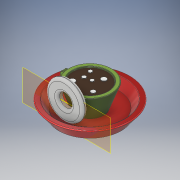
# Autodesk Inventor part: cup
Saved by Autodesk Inventor 2017 (Build 210142000, 142)
## iProperties
Created: 2018-09-11
Part Number: cup
Material: Generic
Document SubType Name: Modeling
Designer: qthuynh
Density: 1 g/cm^3
Appearance: Default
Author: qthuynh
Autodesk Inventor part; units mm, degrees
ref_plane "YZ Plane" through (0, 0, 0) normal (1, 0, 0) x (0, 1, 0)
sketch "Sketch1" plane through (0, 0, 0) normal (0, 0, 1) x (1, 0, 0)
  line L0 (0, 0) -> (0, 101.6)
  line L1 (0, 101.6) -> (61.7893, 101.6)
  line L2 (61.7893, 101.6) -> (88.5597, 137.6833)
  line L3 (88.5597, 137.6833) -> (109.1155, 137.6833)
  line L4 (109.1155, 137.6833) -> (67.5258, 23.4311)
  line L5 (67.5258, 23.4311) -> (143.0565, 23.4311)
  line L6 (143.0565, 23.4311) -> (172.2256, 62.7476)
  line L7 (172.2256, 62.7476) -> (199.4655, 62.7476)
  line L8 (199.4655, 62.7476) -> (152.9127, 0)
  line L9 (152.9127, 0) -> (0, 0)
  dimension "d0" = 101.6
  constraints: 20 end point, 6 parallel, 1 perpendicular, 1 vertical
  measures "d0" distance of L0.start L0.end
revolve "Revolution1" add sketch "Sketch1" angle 360 about axis through (0, 0, 0) along (0, 1, 0)
fillet "Fillet1" radius 3.175 5 edges at (-172.2256, 62.7476, 0) (-152.9127, 0, 0) (-199.4655, 62.7476, 0) (-109.1155, 137.6833, 0) (-88.5597, 137.6833, 0)
ref_plane "Work Plane2" through (0, 0, 0) normal (0, 0, 1) x (1, 0, 0)
sketch "Sketch5" plane through (0, 0, 0) normal (0, 0, 1) x (1, 0, 0)
  ellipse E0 centre (-83.3046, 79.9703) end of major axis (-133.0665, 118.4759) minor radius 30.4237
  ellipse E1 centre (-83.3046, 79.9703) end of major axis (-114.3425, 103.9873) minor radius 19.8321
  point P0 (0, 0)
  constraints: 1 coincident, 4 other
extrude "Extrusion2" add sketch "Sketch5" along normal mid plane 25.4
fillet "Fillet2" radius 3.175 8 edges at (-121.3784, 124.9012, 12.7) (-123.4885, 77.2986, 12.7) (-121.3784, 124.9012, -12.7) (-123.4885, 77.2986, -12.7) (-107.6722, 108.0804, 12.7) (-109.1356, 78.1235, 12.7) (-107.6722, 108.0804, -12.7) (-109.1356, 78.1235, -12.7)
ref_plane "Work Plane3" through (0, 133.35, 0) normal (0, 1, 0) x (-1, 0, 0)
sketch "Sketch6" plane through (0, 133.35, 0) normal (0, 1, 0) x (-1, 0, 0)
  circle A0 centre (0, 0) radius 85.3371
  constraints: 1 centre point, 1 coincident
extrude "Extrusion3" add sketch "Sketch6" against normal blind 25.4
ref_plane "Work Plane4" through (0, 133.35, 0) normal (0, 1, 0) x (-1, 0, 0)
sketch "Sketch7" plane through (0, 133.35, 0) normal (0, 1, 0) x (-1, 0, 0)
  arc A0 (61.639, 4.3067) -> (61.639, -4.3067) centre (0, 0) ccw projected
  circle A1 centre (42.8267, -44.5398) radius 9.1121
  circle A2 centre (-23.9286, -44.5398) radius 12.2561
  circle A3 centre (0, -10.5053) radius 8.7544
  circle A4 centre (-50.6999, 35.319) radius 10.5028
  circle A5 centre (46.5012, 40.6885) radius 13.8683
  circle A6 centre (33.7146, -4.3067) radius 9.6926
  constraints: 6 centre point, 3 point on circle
extrude "Extrusion4" add sketch "Sketch7" along normal blind 2.54
fillet "Fillet3" radius 0.508 7 edges at (-24.022, 135.89, -4.3067) (-32.6329, 135.89, 40.6885) (-32.6329, 133.35, 40.6885) (-33.7146, 135.89, -44.5398) (8.7544, 135.89, -10.5053) (36.1847, 133.35, -44.5398) (61.2027, 133.35, 35.319)
ref_plane "Work Plane5" through (0, 0, 114.3) normal (0, 0, 1) x (1, 0, 0)
sketch "Sketch8" plane through (0, 0, 114.3) normal (0, 0, 1) x (1, 0, 0)
  point P0 (0, 0)
sketch "Sketch10" plane through (0, 0, 114.3) normal (0, 0, 1) x (1, 0, 0)
  line L0 (-61.639, 101.6) -> (61.7893, 101.6) projected
  point P0 (0, 0)
sketch "Sketch11" plane through (0, 0, 114.3) normal (0, 0, 1) x (1, 0, 0)
  circle A0 centre (0, 114.3183) radius 89.777
  circle A1 centre (0, 114.3183) radius 33.623
  point P0 (0, 0)
  constraints: 2 centre point, 1 coincident
extrude "Extrusion6" add sketch "Sketch11" along normal mid plane 27.94
fillet "Fillet5" radius 12.7 3 edges at (-89.777, 114.3183, 100.33) (-89.777, 114.3183, 128.27) (-33.623, 114.3183, 128.27)
body "Solid1"
